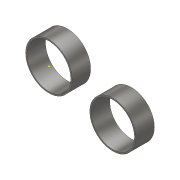
# Autodesk Inventor part: rings
Saved by Autodesk Inventor 2019 (Build 230136000, 136)
## iProperties
Created: 2020-02-18
Part Number: rings
Material: Steel, Cast
Document SubType Name: Modeling
Designer: Admin
Density: 7.85 g/cm^3
Appearance: Semi-Polished
Author: Admin
Autodesk Inventor part; units mm, degrees
ref_plane "YZ Plane" through (0, 0, 0) normal (1, 0, 0) x (0, 1, 0)
ref_plane "XZ Plane" through (0, 0, 0) normal (0, 1, 0) x (-1, 0, 0)
ref_plane "XY Plane" through (0, 0, 0) normal (0, 0, 1) x (1, 0, 0)
sketch "Sketch1" plane through (0, 0, 0) normal (0, 0, 1) x (1, 0, 0)
  circle A0 centre (0, 0) radius 0.4766
  constraints: 1 centre point, 1 coincident
extrude "Extrusion1" add sketch "Sketch1" along normal blind 0.381
sketch "Sketch2" plane through (0, 0, 0.381) normal (0, 0, 1) x (1, 0, 0)
  circle A0 centre (0, 0) radius 0.45
  constraints: 1 centre point, 1 coincident
extrude "Extrusion2" cut sketch "Sketch2" against normal blind 0.381
sketch "Sketch3" plane through (0, 0, 0.381) normal (0, 0, 1) x (1, 0, 0)
  point P0 (0, 0)
sketch "Sketch4" plane through (0, 0, 0.381) normal (0, 0, 1) x (1, 0, 0)
  circle A0 centre (1.6937, 0) radius 0.4723
  point P0 (0, 0)
  constraints: 1 centre point
extrude "Extrusion3" add sketch "Sketch4" along normal blind 0.381
sketch "Sketch5" plane through (1.6937, 0, 0.762) normal (0, 0, 1) x (1, 0, 0)
  circle A0 centre (0, 0) radius 0.4445
  point P0 (-1.6937, 0)
  dimension "d6" = 0.889
  constraints: 1 centre point
  measures "d6" diameter of A0
extrude "Extrusion4" cut sketch "Sketch5" against normal blind 0.381
body "Solid1"
